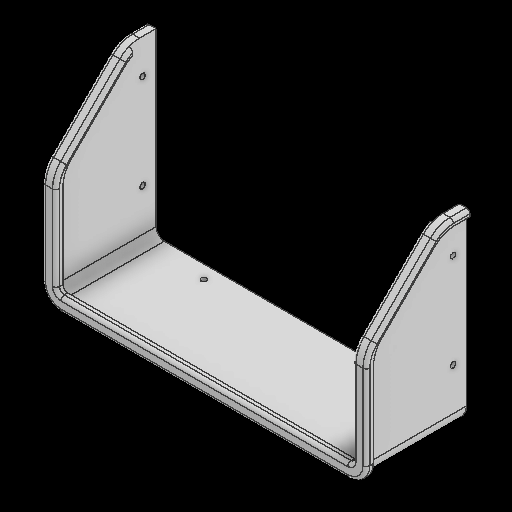
# Autodesk Inventor part: TouchScreen-Bosunre-BO-OFT-080TM-P
Saved by Autodesk Inventor 2025.2 (Build 292293000, 293)
## iProperties
Created: 2026-06-25
Part Number: TouchScreen-Bosunre-BO-OFT-080TM-P
Material: Generic
Document SubType Name: Modeling
Designer: valer
Density: 1 g/cm^3
Appearance: Default
Author: valer
Autodesk Inventor part; units mm, degrees
ref_plane "YZ Plane" through (0, 0, 0) normal (1, 0, 0) x (0, 1, 0)
ref_plane "XZ Plane" through (0, 0, 0) normal (0, 1, 0) x (-1, 0, 0)
ref_plane "XY Plane" through (0, 0, 0) normal (0, 0, 1) x (1, 0, 0)
sketch "Sketch1" plane through (0, 0, 0) normal (0, 0, 1) x (1, 0, 0)
  line L0 (-109, -70.4) -> (109, -70.4)
  line L1 (109, -70.4) -> (109, 70.4)
  line L2 (109, 70.4) -> (-109, 70.4)
  line L3 (-109, 70.4) -> (-109, -70.4)
  line L4 (-109, -70.4) -> (109, 70.4) construction
  line L5 (109, -70.4) -> (-109, 70.4) construction
  point P0 (0, 0)
  dimension "d0" = 218
  dimension "d1" = 140.8
  constraints: 12 end point, 2 midpoint, 2 parallel, 1 horizontal, 1 perpendicular
  measures "d0" distance of L1.end L2.end
  measures "d1" distance of L0.end L1.end
extrude "Extrusion1" add sketch "Sketch1" along normal blind 19.4
sketch "Sketch2" plane through (0, 0, 0) normal (0, 0, -1) x (-1, 0, 0)
  line L0 (109, 70.4) -> (109, -70.4)
  line L1 (-109, -52.169164) -> (109, -52.169164)
  line L2 (109, -52.169164) -> (109, 52.169164)
  line L3 (109, 52.169164) -> (-109, 52.169164)
  line L4 (-109, 52.169164) -> (-109, -52.169164)
  line L5 (-109, -52.169164) -> (109, 52.169164) construction
  line L6 (109, -52.169164) -> (-109, 52.169164) construction
  point P0 (0, 0)
  constraints: 12 end point, 2 midpoint, 2 parallel, 1 horizontal, 1 perpendicular, 1 point on line
extrude "Extrusion2" add sketch "Sketch2" along normal blind 21.8
sketch "Sketch3" plane through (-109, 70.4, 0) normal (0, 1, 0) x (1, 0, 0)
  line L0 (0, 0) -> (0, -19.4) projected
  line L1 (0, -9.7) -> (218, -9.7)
  line L2 (218, 0) -> (218, -19.4) projected
  line L3 (109, 0) -> (109, -19.4)
  line L4 (218, -19.4) -> (0, -19.4) projected
  circle A0 centre (174, -9.7) radius 2
  circle A1 centre (44, -9.7) radius 2
  dimension "d7" = 130
  dimension "d8" = 4
  constraints: 4 end point, 3 midpoint, 2 centre point, 1 point on line, 1 symmetric about line, 1 other
  measures "d7" distance of A0.centre A1.centre
  measures "d8" diameter of A0
extrude "Extrusion3" cut sketch "Sketch3" against normal through all contours A1 L1 | L1 A1 | A0 L1 | L1 A0
sketch "Sketch4" plane through (-109, -70.4, 19.4) normal (-1, 0, 0) x (0, 0, 1)
  line L0 (-19.4, 140.8) -> (0, 140.8) projected
  line L1 (-9.7, 140.8) -> (-9.7, 0)
  line L2 (-19.4, 0) -> (0, 0) projected
  line L3 (-19.4, 70.4) -> (0, 70.4)
  line L4 (0, 140.8) -> (0, 0) projected
  circle A0 centre (-9.7, 104.4) radius 2
  circle A1 centre (-9.7, 36.4) radius 2
  dimension "d11" = 4
  dimension "d12" = 68
  constraints: 4 end point, 3 midpoint, 2 centre point, 1 point on line, 1 symmetric about line, 1 other
  measures "d11" diameter of A0
  measures "d12" distance of A1.centre A0.centre
extrude "Extrusion4" cut sketch "Sketch4" against normal through all contours A0 L1 | L1 A0 | A1 L1 | L1 A1
fillet "Fillet1" radius 6 4 edges at (-109, 70.4, 9.7) (109, 70.4, 9.7) (-109, -70.4, 9.7) (109, -70.4, 9.7)
sketch "Sketch5" plane through (0, 0, 19.4) normal (0, 0, 1) x (1, 0, 0)
  line L0 (-89, -50.4) -> (89, -50.4)
  line L1 (89, -50.4) -> (89, 50.4)
  line L2 (89, 50.4) -> (-89, 50.4)
  line L3 (-89, 50.4) -> (-89, -50.4)
  line L4 (-89, -50.4) -> (89, 50.4) construction
  line L5 (89, -50.4) -> (-89, 50.4) construction
  line L6 (103, 70.4) -> (-103, 70.4) projected
  line L7 (-109, 64.4) -> (-109, -64.4) projected
  point P0 (0, 0)
  dimension "d15" = 20
  dimension "d16" = 20
  constraints: 12 end point, 2 midpoint, 2 parallel, 1 horizontal, 1 perpendicular
  measures "d15" distance between parallel lines of L2 L6
  measures "d16" distance between parallel lines of L7 L3
extrude "Extrusion5" cut sketch "Sketch5" against normal blind 0.5
fillet "Fillet2" radius 6 4 edges at (-109, 52.1692, -10.9) (-109, -52.1692, -10.9) (109, 52.1692, -10.9) (109, -52.1692, -10.9)
sketch "HoodProfile" plane through (0, 0, 19.4) normal (0, 0, 1) x (1, 0, 0)
  line L0 (-89, 50.4) -> (89, 50.4) projected
  line L1 (89, 50.4) -> (89, -50.4) projected
  line L2 (89, -50.4) -> (-89, -50.4) projected
  line L3 (-89, -50.4) -> (-89, 50.4) projected
  arc A0 (103, -70.4) -> (109, -64.4) centre (103, -64.4) ccw projected
  line L4 (109, -64.4) -> (109, 64.4) projected
  arc A1 (109, 64.4) -> (103, 70.4) centre (103, 64.4) ccw projected
  line L5 (103, 70.4) -> (-103, 70.4) projected
  arc A2 (-103, 70.4) -> (-109, 64.4) centre (-103, 64.4) ccw projected
  line L6 (-109, 64.4) -> (-109, -64.4) projected
  arc A3 (-109, -64.4) -> (-103, -70.4) centre (-103, -64.4) ccw projected
  line L7 (-103, -70.4) -> (103, -70.4) projected
  arc A4 (103, -75.4) -> (114, -64.4) centre (103, -64.4) ccw
  line L8 (114, -64.4) -> (114, 64.4)
  arc A5 (114, 64.4) -> (103, 75.4) centre (103, 64.4) ccw
  line L9 (103, 75.4) -> (-103, 75.4)
  arc A6 (-103, 75.4) -> (-114, 64.4) centre (-103, 64.4) ccw
  line L10 (-114, 64.4) -> (-114, -64.4)
  arc A7 (-114, -64.4) -> (-103, -75.4) centre (-103, -64.4) ccw
  line L11 (-103, -75.4) -> (103, -75.4)
  line L12 (114, 54.6) -> (-114, 54.6)
  point P0 (0, 0)
  point P1 (-109, 54.6)
  point P2 (109, 54.6)
  dimension "d20" = 5
  dimension "d21" = 150.8
  dimension "d22" = 130
  constraints: 10 end point, 8 point on circle, 4 centre point, 2 point on line, 1 perpendicular, 7 other
  measures "d20" distance between parallel lines of L7 L11
  measures "d21" distance between parallel lines of L9 L11
  measures "d22" distance between parallel lines of L11 L12
extrude "HoodFeature" add sketch "HoodProfile" along normal blind 50 separate body contours A0 L4 L12 L8 A4 L11 A7 L10 L6 A3 L7
sketch "HoodDraft" plane through (114, -64.4, 19.4) normal (1, 0, 0) x (0, 0, -1)
  line L0 (-50, 119) -> (-50, 0) projected
  line L1 (-50, 69) -> (0, 119)
  line L2 (0, 119) -> (-50, 119) projected
  point P0 (19.4, 64.4)
  dimension "d7" = 130
  dimension "d8" = 4
  dimension "d25" = 45
  constraints: 2 end point, 1 point on line
  measures "d25" angle of L0 L1
extrude "HoodDraftFeature" cut sketch "HoodDraft" against normal through all bodies 2
sketch "Sketch8" plane through (0, 0, 19.4) normal (0, 0, -1) x (-1, 0, 0)
  line L0 (-103, -70.4) -> (103, -70.4) projected
  arc A0 (-109, -64.4) -> (-103, -70.4) centre (-103, -64.4) ccw projected
  line L1 (-109, 54.6) -> (-109, -64.4) projected
  line L2 (-114, 54.6) -> (-109, 54.6) projected
  line L3 (-114, -64.4) -> (-114, 54.6) projected
  arc A1 (-114, -64.4) -> (-103, -75.4) centre (-103, -64.4) ccw projected
  line L4 (103, -75.4) -> (-103, -75.4) projected
  arc A2 (103, -75.4) -> (114, -64.4) centre (103, -64.4) ccw projected
  line L5 (114, 54.6) -> (114, -64.4) projected
  line L6 (109, 54.6) -> (114, 54.6) projected
  line L7 (109, -64.4) -> (109, 54.6) projected
  arc A3 (103, -70.4) -> (109, -64.4) centre (103, -64.4) ccw projected
  point P0 (0, 0)
extrude "Extrusion8" add sketch "Sketch8" along normal up to surface (19.4 mm away) bodies 2
sketch "Sketch9" plane through (114, -64.4, 69.4) normal (1, 0, 0) x (0, 0, -1)
  circle A0 centre (59.7, 30.4) radius 2 projected
  circle A1 centre (59.7, 98.4) radius 2 projected
  point P0 (69.4, 64.4)
extrude "Extrusion9" cut sketch "Sketch9" against normal through all bodies 2
sketch "Sketch10" plane through (-103, -75.4, 69.4) normal (0, -1, 0) x (1, 0, 0)
  circle A0 centre (38, -59.7) radius 2 projected
  circle A1 centre (168, -59.7) radius 2 projected
  point P0 (103, -69.4)
extrude "Extrusion10" cut sketch "Sketch10" against normal blind 10 bodies 2
sketch "Sketch11" plane through (0, 0, 69.4) normal (0, 0, 1) x (1, 0, 0)
  line L0 (109, 4.6) -> (109, -64.4) projected
  arc A0 (103, -70.4) -> (109, -64.4) centre (103, -64.4) ccw projected
  line L1 (103, -70.4) -> (-103, -70.4) projected
  arc A1 (-109, -64.4) -> (-103, -70.4) centre (-103, -64.4) ccw projected
  line L2 (-109, -64.4) -> (-109, 4.6) projected
  line L3 (-114, 4.6) -> (-114, -64.4) projected
  arc A2 (-114, -64.4) -> (-103, -75.4) centre (-103, -64.4) ccw projected
  line L4 (-103, -75.4) -> (103, -75.4) projected
  arc A3 (103, -75.4) -> (114, -64.4) centre (103, -64.4) ccw projected
  line L5 (114, -64.4) -> (114, 4.6) projected
  line L6 (103, -77.9) -> (-103, -77.9)
  arc A4 (-116.5, -64.4) -> (-103, -77.9) centre (-103, -64.4) ccw
  line L7 (-116.5, -64.4) -> (-116.5, 4.6)
  line L8 (-116.5, 4.6) -> (-106.5, 4.6)
  line L9 (-106.5, 4.6) -> (-106.5, -64.4)
  arc A5 (-106.5, -64.4) -> (-103, -67.9) centre (-103, -64.4) ccw
  line L10 (-103, -67.9) -> (103, -67.9)
  arc A6 (103, -67.9) -> (106.5, -64.4) centre (103, -64.4) ccw
  line L11 (106.5, -64.4) -> (106.5, 4.6)
  line L12 (106.5, 4.6) -> (116.5, 4.6)
  line L13 (116.5, 4.6) -> (116.5, -64.4)
  arc A7 (103, -77.9) -> (116.5, -64.4) centre (103, -64.4) ccw
  line L14 (114, 4.6) -> (109, 4.6) projected
  line L15 (-109, 4.6) -> (-114, 4.6) projected
  line L16 (114, 4.6) -> (109, 4.6) projected
  point P0 (0, 0)
  dimension "d36" = 2.5
  dimension "d56" = 2.5
  dimension "d57" = 2.5
  constraints: 16 end point, 8 point on circle, 4 centre point, 2 collinear, 7 other
  measures "d36" distance between parallel lines of L4 L6
  measures "d56" radial gap between concentric circles of A7 A3
  measures "d57" distance between parallel lines of L2 L9
extrude "Extrusion11" add sketch "Sketch11" along normal blind 5 bodies 2
sketch "Sketch12" plane through (109, 4.6, 69.4) normal (0, 0.7071068, 0.7071068) x (1, 0, 0)
  line L0 (0, 0) -> (0, 70.710678)
  line L1 (5, 70.710678) -> (5, 0)
  line L2 (5, 70.710678) -> (0, 70.710678)
  line L3 (-218, 70.710678) -> (-218, 8.284271)
  line L4 (-218, 70.710678) -> (-218, 0)
  line L5 (-218, 70.710678) -> (-223, 70.710678)
  line L6 (-223, 0) -> (-223, 70.710678)
  line L7 (7.5, -2.5) -> (-2.5, -2.5)
  line L8 (-2.5, -2.5) -> (-2.5, 73.210678)
  line L9 (-2.5, 73.210678) -> (7.5, 73.210678)
  line L10 (7.5, 73.210678) -> (7.5, -2.5)
  line L11 (-225.5, 73.210678) -> (-215.5, 73.210678)
  line L12 (-215.5, 73.210678) -> (-215.5, -2.5)
  line L13 (-215.5, -2.5) -> (-225.5, -2.5)
  line L14 (-225.5, -2.5) -> (-225.5, 73.210678)
  line L15 (5, 0) -> (0, 0)
  line L16 (-218, 0) -> (-223, 0)
  point P0 (-109, 45.820519)
  dimension "d39" = 2.5
  dimension "d40" = 2.5
  constraints: 16 end point, 3 other
  measures "d39" distance between parallel lines of L1 L10
  measures "d40" distance between parallel lines of L6 L14
extrude "Extrusion12" add sketch "Sketch12" along normal up to surface (3.535534 mm away) contours L0 L2 L1 L15 | L3 L4 L16 L6 L5 | L7 L8 L9 L10 | L11 L12 L13 L14 bodies 2
sketch "Sketch13" plane through (109, 54.6, 0) normal (0, 1, 0) x (1, 0, 0)
  line L0 (0, 0) -> (5, 0) projected
  line L1 (0, -19.4) -> (0, 0) projected
  line L2 (5, -19.4) -> (0, -19.4) projected
  line L3 (5, -19.4) -> (5, 0) projected
  line L4 (-223, 0) -> (-218, 0) projected
  line L5 (-223, -19.4) -> (-223, 0) projected
  line L6 (-218, -19.4) -> (-223, -19.4) projected
  line L7 (-218, -19.4) -> (-218, 0) projected
  line L8 (7.5, 2.5) -> (-2.5, 2.5)
  line L9 (-2.5, 2.5) -> (-2.5, -21.9)
  line L10 (-2.5, -21.9) -> (7.5, -21.9)
  line L11 (7.5, -21.9) -> (7.5, 2.5)
  line L12 (-225.5, 2.5) -> (-215.5, 2.5)
  line L13 (-215.5, 2.5) -> (-215.5, -21.9)
  line L14 (-215.5, -21.9) -> (-225.5, -21.9)
  line L15 (-225.5, -21.9) -> (-225.5, 2.5)
  point P0 (-109, 0)
  dimension "d43" = 2.5
  dimension "d44" = 2.5
  constraints: 16 end point, 6 other
  measures "d43" distance between parallel lines of L3 L11
  measures "d44" distance between parallel lines of L5 L15
extrude "Extrusion13" add sketch "Sketch13" along normal up to surface (4.267767 mm away) contours L0 L3 L2 L1 | L4 L7 L6 L5 | L11 L10 L9 L8 | L12 L13 L14 L15 bodies 2
delete faces "Delete1" heal yes whole lump no faces at (109.833333, 4.844078, 73.179612) (-113.166667, 4.844078, 73.179612)
delete faces "Delete2" heal yes whole lump no faces at (-109.833333, 57.689256, 21.9) (113.166667, 57.689256, 21.9)
fillet "Fillet5" radius 20 12 edges at (111.5, 4.6, 74.4) (-111.5, 4.6, 74.4) (111.5, 58.8678, 20.1322) (-111.5, 58.8678, 20.1322) (115.25, 54.6, 19.4) (115.25, 4.6, 69.4) (-115.25, 4.6, 69.4) (-115.25, 54.6, 19.4) (-107.75, 4.6, 69.4) (-107.75, 54.6, 19.4) (107.75, 4.6, 69.4) (107.75, 54.6, 19.4)
fillet "Fillet6" radius 2.5 26 edges at (116.5, -34.0421, 74.4) (116.5, 3.9694, 72.8776) (116.5, 31.7339, 47.2661) (116.5, 57.3454, 19.5016) (116.5, 58.8678, 4.674) (0, -77.9, 74.4) (-112.5459, -73.9459, 74.4) (-116.5, -34.0421, 74.4) (-116.5, 3.9694, 72.8776) (-116.5, 31.7339, 47.2661) (-116.5, 57.3454, 19.5016) (-116.5, 58.8678, 4.674) (112.5459, -73.9459, 74.4) (-106.5, -34.0421, 74.4) (-106.5, 3.9694, 72.8776) (-106.5, 31.7339, 47.2661) (-106.5, 57.3454, 19.5016) (-106.5, 58.8678, 4.674) (0, -67.9, 74.4) (105.4749, -66.8749, 74.4) (106.5, -34.0421, 74.4) (106.5, 3.9694, 72.8776) (106.5, 31.7339, 47.2661) (106.5, 57.3454, 19.5016) (106.5, 58.8678, 4.674) (-105.4749, -66.8749, 74.4)
fillet "Fillet8" radius 1.8 13 edges at (110.7782, -72.1782, 69.4) (114, -34.0421, 69.4) (114, 3.9694, 67.8776) (114, 29.6, 44.4) (114, 53.0776, 18.7694) (114, 54.6, 5.5579) (-110.7782, -72.1782, 69.4) (-114, -34.0421, 69.4) (-114, 3.9694, 67.8776) (-114, 29.6, 44.4) (-114, 53.0776, 18.7694) (-114, 54.6, 5.5579) (0, -75.4, 69.4)
fillet "Fillet9" radius 1.8 13 edges at (-107.2426, -68.6426, 69.4) (-109, -34.0421, 69.4) (-109, 3.9694, 67.8776) (-109, 29.6, 44.4) (-109, 53.0776, 18.7694) (-109, 54.6, 5.5579) (107.2426, -68.6426, 69.4) (109, -34.0421, 69.4) (109, 3.9694, 67.8776) (109, 29.6, 44.4) (109, 53.0776, 18.7694) (109, 54.6, 5.5579) (0, -70.4, 69.4)
split "Sculpt1" plane through (103, -75.4, 0) removes the side toward (0, 0, -1) bodies 2
ref_plane "Work Plane1" through (103, -75.4, 0) normal (0, 0, -1) x (-1, 0, 0)
sketch "Sketch14" plane through (109, 58.867767, 0) normal (0, 1, 0) x (1, 0, 0)
  line L0 (0, -19.4) -> (0, 0) projected
  line L1 (-218, 0) -> (-218, -19.4) projected
  line L2 (-218, -19.4) -> (0, -19.4)
  line L3 (0, -19.4) -> (0, 0)
  line L4 (0, 0) -> (-2.5, 0) projected
  line L5 (0, 0) -> (-218, 0)
  point P0 (-109, 0)
  point P1 (-2.5, 0)
  constraints: 6 end point, 2 perpendicular, 1 collinear
extrude "Extrusion14" cut sketch "Sketch14" against normal blind 50 bodies 2
equation "\"d56\" = d36"
equation "\"d57\" = d36"
